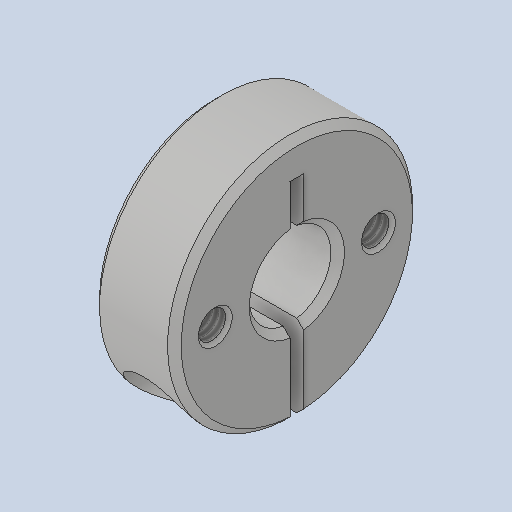
# Autodesk Inventor part: SCSWJ6-6_b
Saved by Autodesk Inventor 2025.1 (Build 291241000, 241)
## iProperties
Category: PARTsolutions
Company: MISUMI
Created: 2024-03-18
Part Number: SCSWJ6-6_b
Material: Generic
Catalog Web Link: www.cadenas.de
Description: SCSWJ, PSCSWJ, SSCSWJ_b-Set Collars - Slit 2 Hole/2 Tap - Compact Type - 2 Tap Type
Vendor: MISUMI
Document SubType Name: Modeling
Designer: psAdmin
Manufacturer: MISUMI
Mass: 1.14086 g
Surface Area: 10.8581 cm^2
Volume: 1.14086 cm^3
Density: 1 g/cm^3
Appearance: PSOLRGB-175-175-175
PSOL_IDENT_0: {$CADENAS_DATA/23d-libs/misumi/metric/03_set_collars/scswj/scswj_b.prj},182 {VTYP=3D},{NB=SCSWJ6-6_b
PSOL_IDENT_1: },{LINA=SCSWJ6-6},{NN=SCSWJ, PSCSWJ, SSCSWJ_b},{DATE=30.11.2021 05:42:06},{GEOMDATE=24.09.2021 04:03
PSOL_IDENT_2: :07},{VERSION=},{LINEID=220},{WBVAR=MAT,ST},{WBNUMERIC=}  {NB=SCSWJ6-6_b},{LINA=SCSWJ6-6},{KT=DUMMY}
PSOL_IDENT_3: ,{PN=SCSWJ6-6},{TYPE=SCSWJ},{MAT=1045},{MATA='1045','S45C Equivalent','304','SUS304 Equivalent'},{ST=
PSOL_IDENT_4: BO},{ST0='BO','Black Oxide','ENP','Electroless Nickel Plating'},{AC=Hexagon Socket Head Set Screw 1
PSOL_IDENT_5: Pc.},{D=6},{B=6},{D1=18},{M=M2.5},{THMD=2.5},{THDMIN=2.013},{DD=2.9},{R=2.45},{W=1.0},{X=6.0},{Y=3},
PSOL_IDENT_6: {Z=6.5},{P=12},{C=0.5},{L=6},{M1=M2.5},{THMD1=2.5},{THDMIN1=2.013}
NB: SCSWJ6-6_b
NN: SCSWJ, PSCSWJ, SSCSWJ_b
NT: Set Collars - Slit 2 Hole/2 Tap - Compact Type - 2 Tap Type
NBSYN: $PN._b
LINA: SCSWJ6-6
CATALOG: Misumi
PN: SCSWJ6-6
MAT: S45C Equivalent
ST: Black Oxide
AC: Hexagon Socket Head Set Screw 1 Pc.
D: 6
B: 6
D1: 18
M: M2.5
DD: 2.9
R: 2.45
W: 1
X: 6
Y: 3
Z: 6.5
P: 12
M1: M2.5
SUPPLIER: MISUMI
ARTICLENO: SCSWJ6-6_b
BOMINFO: SCSWJ6-6
CREATOR: CADENAS GmbH
d13: 0.000 mm
Title: SCSWJ6-6
Author: Cadenas PARTsolutions
Comments: Set Collars - Slit 2 Hole/2 Tap - Compact Type - 2 Tap Type
Autodesk Inventor part; units mm, degrees
sketch "Sketch_1" plane through (0, 0, 0) normal (0, 0, 1) x (1, 0, 0)
  line L0 (3, 0) -> (-3, 0)
  line L1 (-3, 8.5) -> (-3, 3.5)
  line L2 (-3, 3.5) -> (-2.5, 3)
  line L3 (-2.5, 3) -> (2.5, 3)
  line L4 (2.5, 3) -> (3, 3.5)
  line L5 (3, 3.5) -> (3, 8.5)
  line L6 (3, 8.5) -> (2.5, 9)
  line L7 (2.5, 9) -> (-2.5, 9)
  line L8 (-2.5, 9) -> (-3, 8.5)
  constraints: 18 end point
revolve "Revolution1" add sketch "Sketch_1" angle 360 about axis through (3, 0, 0) along (1, 0, 0)
sketch "Sketch_2" plane through (0, 0, 0) normal (1, 0, 0) x (0, 1, 0)
  line L0 (-9, 0.5) -> (-9, -0.5)
  line L1 (-9, -0.5) -> (6.5, -0.5)
  line L2 (6.5, -0.5) -> (6.5, 0.5)
  line L3 (6.5, 0.5) -> (-9, 0.5)
  constraints: 8 end point
extrude "Extrusion1" cut sketch "Sketch_2" along normal mid plane 6
sketch "Sketch_3" plane through (0, 0, 0) normal (1, 0, 0) x (0, 1, 0)
  line L0 (-6, 9) -> (-6, 0)
  line L1 (-6, 0) -> (-7.45, 0)
  line L2 (-7.45, 0) -> (-7.45, 3)
  line L3 (-7.45, 3) -> (-8.45, 3)
  line L4 (-8.45, 3) -> (-8.45, 9)
  line L5 (-8.45, 9) -> (-6, 9)
  line L6 (-6, 9) -> (-6, 0)
  constraints: 14 end point
revolve "Revolution2" cut sketch "Sketch_3" angle 360 about axis through (0, -6, 9) along (0, 0, 1)
sketch "Sketch_4" plane through (0, 0, 0) normal (1, 0, 0) x (0, 1, 0)
  line L0 (-6, -9.5) -> (-6, -0.5)
  line L1 (-6, -0.5) -> (-4.75, -0.5)
  line L2 (-4.75, -0.5) -> (-4.9935, -0.7435)
  line L3 (-4.9935, -0.7435) -> (-4.9935, -9.5)
  line L4 (-4.9935, -9.5) -> (-6, -9.5)
  line L5 (-6, -9.5) -> (-6, -0.5)
  constraints: 12 end point
revolve "Revolution3" cut sketch "Sketch_4" angle 360 about axis through (0, -6, -9.5) along (0, 0, -1)
thread "Thread1" size "M2.5x0.45" class "6H" standard "ISO Metric profile" length 6.9009
sketch "Sketch_7" plane through (0, 0, -6) normal (0, 0, 1) x (1, 0, 0)
  line L0 (3, 0) -> (-3, 0)
  line L1 (-3, 0) -> (-3, 1.25)
  line L2 (-3, 1.25) -> (-2.7565, 1.0065)
  line L3 (-2.7565, 1.0065) -> (2.7565, 1.0065)
  line L4 (2.7565, 1.0065) -> (3, 1.25)
  line L5 (3, 1.25) -> (3, 0)
  line L6 (3, 0) -> (-3, 0)
  constraints: 14 end point
revolve "Revolution4" cut sketch "Sketch_7" angle 360 about axis through (3, 0, -6) along (1, 0, 0)
thread "Thread2" size "M2.5x0.45" class "6H" standard "ISO Metric profile" full length
sketch "Sketch_8" plane through (0, 0, 6) normal (0, 0, 1) x (1, 0, 0)
  line L0 (3, 0) -> (-3, 0)
  line L1 (-3, 0) -> (-3, 1.25)
  line L2 (-3, 1.25) -> (-2.7565, 1.0065)
  line L3 (-2.7565, 1.0065) -> (2.7565, 1.0065)
  line L4 (2.7565, 1.0065) -> (3, 1.25)
  line L5 (3, 1.25) -> (3, 0)
  line L6 (3, 0) -> (-3, 0)
  constraints: 14 end point
revolve "Revolution5" cut sketch "Sketch_8" angle 360 about axis through (3, 0, 6) along (1, 0, 0)
thread "Thread3" size "M2.5x0.45" class "6H" standard "ISO Metric profile" full length
ref_plane "body_screw_XY" through (0, -6, 3) normal (0, 0, 1) x (1, 0, 0)
ref_plane "body_screw_YZ" through (0, -6, 3) normal (1, 0, 0) x (0, 1, 0)
ref_plane "body_screw_ZX" through (0, -6, 3) normal (0, 1, 0) x (0, 0, 1)
body "Solid1"
